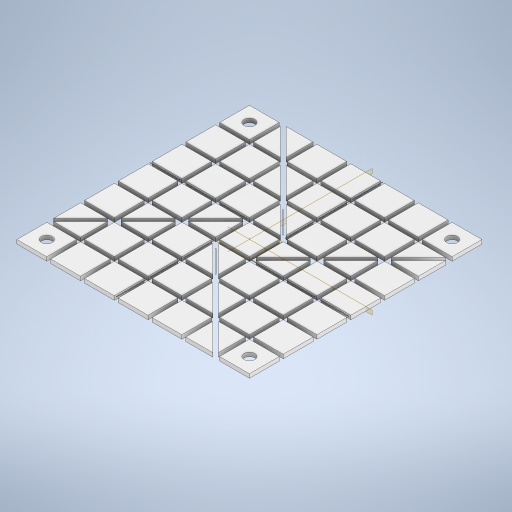
# Autodesk Inventor part: Flasher2
Saved by Autodesk Inventor 2024 (Build 280153000, 153)
## iProperties
Created: 2023-02-28
Part Number: Flasher2
Material: ABS Plastic
Document SubType Name: Modeling
Designer: byrne
Density: 1.06 g/cm^3
Appearance: Smooth - White
Author: byrne
Autodesk Inventor part; units mm, degrees
ref_plane "YZ Plane" through (0, 0, 0) normal (1, 0, 0) x (0, 1, 0)
ref_plane "XZ Plane" through (0, 0, 0) normal (0, 1, 0) x (-1, 0, 0)
ref_plane "XY Plane" through (0, 0, 0) normal (0, 0, 1) x (1, 0, 0)
sketch "Sketch1" plane through (0, 0, 0) normal (0, 1, 0) x (-1, 0, 0)
  line L0 (0, 0) -> (95.25, 0) construction
  line L1 (95.25, 0) -> (95.25, -95.25) construction
  line L2 (95.25, -95.25) -> (0, -95.25)
  line L3 (0, -95.25) -> (0, 0)
  line L4 (54.4286, -40.8214) -> (40.8214, -40.8214)
  line L5 (40.8214, -40.8214) -> (40.8214, -54.4286)
  line L6 (40.8214, -54.4286) -> (54.4286, -54.4286)
  line L7 (54.4286, -54.4286) -> (54.4286, -40.8214)
  line L8 (54.4286, -54.4286) -> (95.25, -13.6071)
  line L9 (40.8214, -54.4286) -> (81.6429, -95.25)
  line L10 (40.8214, -40.8214) -> (0, -81.6429)
  line L11 (54.4286, -40.8214) -> (13.6071, 0)
  line L12 (40.8214, -40.8214) -> (0, -40.8214)
  line L13 (40.8214, -54.4286) -> (40.8214, -95.25)
  line L14 (54.4286, -54.4286) -> (95.25, -54.4286)
  line L15 (54.4286, -40.8214) -> (54.4286, 0)
  line L16 (81.6429, -13.6071) -> (95.25, -13.6071)
  line L17 (81.6429, -13.6071) -> (81.6429, 0)
  line L18 (81.6429, -81.6429) -> (95.25, -81.6429)
  line L19 (81.6429, -81.6429) -> (81.6429, -95.25)
  line L20 (95.25, -81.6429) -> (95.25, -95.25)
  line L21 (95.25, -95.25) -> (81.6429, -95.25)
  line L22 (95.25, -13.6071) -> (95.25, 0)
  line L23 (95.25, 0) -> (81.6429, 0)
  line L24 (13.6071, 0) -> (0, 0)
  line L25 (0, -13.6071) -> (13.6071, -13.6071)
  line L26 (40.8214, -68.0357) -> (0, -68.0357)
  line L27 (40.8214, -54.4286) -> (0, -54.4286)
  line L28 (13.6071, -40.8214) -> (13.6071, -95.25)
  line L29 (40.8214, -81.6429) -> (0, -81.6429)
  line L30 (27.2143, -40.8214) -> (27.2143, -95.25)
  line L31 (41.3827, -41.3827) -> (1.9163, -80.8491)
  line L32 (1.9163, -80.8491) -> (40.8214, -80.8491)
  line L33 (40.2602, -40.2602) -> (-1.9163, -82.4366)
  line L34 (-1.9163, -82.4366) -> (40.8214, -82.4366)
  line L35 (40.8214, -68.8295) -> (0, -68.8295)
  line L36 (40.8214, -67.242) -> (0, -67.242)
  line L37 (26.4205, -40.8214) -> (26.4205, -95.25)
  line L38 (28.008, -40.8214) -> (28.008, -95.25)
  line L39 (40.0277, -54.4286) -> (40.0277, -95.25)
  line L40 (40.8214, -55.2223) -> (0, -55.2223)
  line L41 (40.8214, -53.6348) -> (0, -53.6348)
  line L42 (40.0277, -40.8214) -> (40.0277, -54.4286)
  line L43 (40.8214, -41.6152) -> (0, -41.6152)
  line L44 (14.4009, -40.8214) -> (14.4009, -95.25)
  line L45 (12.8134, -40.8214) -> (12.8134, -95.25)
  line L46 (0.7938, -95.25) -> (0.7937, -0.7938)
  line L47 (0.7937, -0.7938) -> (13.2784, -0.7938)
  line L48 (13.2784, -0.7938) -> (53.8673, -41.3827)
  line L49 (95.25, -94.4562) -> (0, -94.4562)
  line L50 (54.4286, -41.6152) -> (40.8214, -41.6152)
  line L51 (41.6152, -40.8214) -> (41.6152, -54.4286)
  line L52 (40.8214, -53.6348) -> (54.4286, -53.6348)
  line L53 (53.6348, -54.4286) -> (53.6348, -40.8214)
  circle A0 centre (6.8036, -88.4464) radius 2.159
  point P0 (27.2143, 0)
  point P1 (40.8214, 0)
  point P2 (68.0357, 0)
  point P3 (27.2143, -13.6071)
  point P4 (40.8214, -13.6071)
  point P5 (54.4286, -13.6071)
  point P6 (68.0357, -13.6071)
  point P7 (0, -27.2143)
  point P8 (13.6071, -27.2143)
  point P9 (27.2143, -27.2143)
  point P10 (40.8214, -27.2143)
  point P11 (54.4286, -27.2143)
  point P12 (68.0357, -27.2143)
  point P13 (81.6429, -27.2143)
  point P14 (95.25, -27.2143)
  point P15 (68.0357, -40.8214)
  point P16 (81.6429, -40.8214)
  point P17 (95.25, -40.8214)
  point P18 (13.6071, -54.4286)
  point P19 (27.2143, -54.4286)
  point P20 (68.0357, -54.4286)
  point P21 (81.6429, -54.4286)
  point P22 (13.6071, -68.0357)
  point P23 (27.2143, -68.0357)
  point P24 (54.4286, -68.0357)
  point P25 (68.0357, -68.0357)
  point P26 (81.6429, -68.0357)
  point P27 (95.25, -68.0357)
  point P28 (13.6071, -81.6429)
  point P29 (27.2143, -81.6429)
  point P30 (54.4286, -81.6429)
  point P31 (68.0357, -81.6429)
  point P32 (95.25, -81.6429)
  point P33 (0, -95.25)
  point P34 (54.4286, -95.25)
  point P35 (68.0357, -95.25)
  point P36 (53.6348, -53.6348)
  point P37 (53.6348, -41.6152)
  point P38 (41.6152, -41.6152)
  point P39 (41.6152, -53.6348)
  point P40 (0.7937, -55.2223)
  point P41 (0.7937, -67.242)
  point P42 (12.8134, -67.242)
  point P43 (12.8134, -55.2223)
  point P44 (0.7937, -41.6152)
  point P45 (0.7937, -53.6348)
  point P46 (12.8134, -53.6348)
  point P47 (12.8134, -41.6152)
  point P48 (0.7937, -68.8295)
  point P49 (0.7937, -79.7266)
  point P50 (11.6909, -68.8295)
  point P51 (12.8134, -80.8491)
  point P52 (12.8134, -69.952)
  point P53 (0.7937, -94.4562)
  point P54 (12.8134, -94.4562)
  point P55 (12.8134, -82.4366)
  point P56 (0.7937, -82.4366)
  point P57 (14.4009, -94.4562)
  point P58 (26.4205, -94.4562)
  point P59 (26.4205, -82.4366)
  point P60 (14.4009, -82.4366)
  point P61 (14.4009, -68.8295)
  point P62 (14.4009, -80.8491)
  point P63 (26.4205, -80.8491)
  point P64 (26.4205, -68.8295)
  point P65 (26.4205, -67.242)
  point P66 (26.4205, -56.3449)
  point P67 (15.5234, -67.242)
  point P68 (14.4009, -55.2223)
  point P69 (14.4009, -66.1194)
  point P70 (25.298, -55.2223)
  point P71 (14.4009, -41.6152)
  point P72 (14.4009, -53.6348)
  point P73 (26.4205, -53.6348)
  point P74 (26.4205, -41.6152)
  point P75 (38.9051, -41.6152)
  point P76 (28.008, -41.6152)
  point P77 (28.008, -52.5123)
  point P78 (40.0277, -53.6348)
  point P79 (40.0277, -42.7377)
  point P80 (29.1306, -53.6348)
  point P81 (40.0277, -55.2223)
  point P82 (28.008, -55.2223)
  point P83 (28.008, -67.242)
  point P84 (40.0277, -67.242)
  point P85 (40.0277, -80.8491)
  point P86 (40.0277, -68.8295)
  point P87 (28.008, -68.8295)
  point P88 (28.008, -80.8491)
  point P89 (28.008, -94.4562)
  point P90 (40.0277, -94.4562)
  point P91 (40.0277, -82.4366)
  point P92 (28.008, -82.4366)
  dimension "d0" = 95.25
  dimension "d1" = 95.25
  dimension "d4" = 13.6071
  dimension "d7" = 13.6071
  dimension "d10" = 0.7937
  dimension "d11" = 0.7937
  dimension "d12" = 0.7937
  dimension "d13" = 0.7937
  dimension "d14" = 0.7937
  dimension "d15" = 0.7937
  dimension "d16" = 0.7937
  dimension "d17" = 0.7937
  dimension "d18" = 0.7937
  dimension "d19" = 0.7937
  dimension "d20" = 0.7937
  dimension "d21" = 0.7937
  dimension "d22" = 0.7937
  dimension "d23" = 0.7937
  dimension "d24" = 0.7937
  dimension "d25" = 0.7937
  dimension "d26" = 0.7937
  dimension "d27" = 0.7937
  dimension "d28" = 0.7937
  dimension "d36" = 4.318
  dimension "d37" = 6.8036
  dimension "d38" = 6.8036
  constraints: 108 end point, 20 parallel, 7 horizontal, 6 perpendicular, 6 vertical, 3 collinear, 2 point on line, 1 centre point, 67 other
  measures "d0" distance of L1.end L2.end
  measures "d1" distance of L0.end L1.end
  measures "d4" distance of L0.start L11.end
  measures "d7" distance of L0.start L25.start
  measures "d10" distance between parallel lines of L10 L31
  measures "d11" distance between parallel lines of L10 L33
  measures "d12" distance between parallel lines of L26 L35
  measures "d13" distance between parallel lines of L26 L36
  measures "d14" distance between parallel lines of L30 L37
  measures "d15" distance between parallel lines of L30 L38
  measures "d16" distance between parallel lines of L13 L39
  measures "d17" distance between parallel lines of L27 L40
  measures "d18" distance between parallel lines of L27 L41
  measures "d19" distance between parallel lines of L5 L42
  measures "d20" distance between parallel lines of L12 L43
  measures "d21" distance between parallel lines of L28 L44
  measures "d22" distance between parallel lines of L28 L45
  measures "d23" distance between parallel lines of L3 L46
  measures "d24" distance between parallel lines of L2 L49
  measures "d25" distance between parallel lines of L4 L50
  measures "d26" distance between parallel lines of L5 L51
  measures "d27" distance between parallel lines of L6 L52
  measures "d28" distance between parallel lines of L7 L53
  measures "d36" diameter of A0
  measures "d37" distance from line of L2 A0.centre
  measures "d38" distance from line of A0.centre L3
extrude "Extrusion1" add sketch "Sketch1" along normal blind 1.5875 contours L51 L50 L53 L52
extrude "Extrusion2" add sketch "Sketch1" along normal blind 1.5875 contours L49 L38 L34 L39 | L41 L31 L42 | L39 L36 L38 L40 | L49 L44 L34 L37 | L32 L38 L35 L39 | L33 L38 L43 | L36 L31 L37 | L33 L44 L40 | L49 L46 L34 L45 | L32 L44 L35 L37 | L41 L44 L43 L37 | L33 L46 L35 | L45 L32 L31 | L36 L46 L40 L45 | L41 L46 L43 L45
ref_plane "Work Plane1" through (-47.625, 0, -41.6152) normal (1, 0, 0) x (0, 0, -1)
ref_plane "Work Plane2" through (-53.6348, 0, -47.625) normal (0, 0, 1) x (1, 0, 0)
pattern_circular "Circular Pattern1" count 4 over 360 about axis through (-47.625, 0, -47.625) along (0, -1, 0) of "Extrusion2"
sketch "Sketch3" plane through (0, 1.5875, 0) normal (0, 1, 0) x (1, 0, 0)
  line L0 (-40.9484, 94.3927) -> (-40.6944, 94.3927)
  line L1 (-40.6944, 55.2767) -> (-40.9484, 55.2767)
  line L2 (-41.6152, 94.4563) -> (-53.6348, 94.4563) projected
  line L3 (-40.0277, 94.4562) -> (-40.0277, 82.4366) projected
  line L4 (-41.6152, 94.4563) -> (-40.0277, 94.4562)
  line L5 (-40.9484, 82.4366) -> (-40.6944, 82.4366)
  line L6 (-53.6348, 82.4366) -> (-41.6152, 82.4366) projected
  line L7 (-40.9484, 80.8491) -> (-40.6944, 80.8491)
  line L8 (-41.6152, 80.8491) -> (-53.6348, 80.8491) projected
  line L9 (-40.9484, 68.8295) -> (-40.6944, 68.8295)
  line L10 (-40.9484, 67.242) -> (-40.6944, 67.242)
  line L11 (-53.6348, 68.8295) -> (-41.6152, 68.8295) projected
  line L12 (-41.6152, 67.242) -> (-52.5123, 67.242) projected
  line L13 (-40.6944, 94.3927) -> (-40.6944, 82.4366)
  line L14 (-40.9484, 82.4366) -> (-40.9484, 94.3927)
  line L15 (-40.6944, 80.8491) -> (-40.6944, 68.8295)
  line L16 (-40.6944, 67.242) -> (-40.6944, 55.2767)
  line L17 (-40.9484, 55.2767) -> (-40.9484, 67.242)
  line L18 (-40.9484, 68.8295) -> (-40.9484, 80.8491)
  line L19 (-41.6152, 53.6348) -> (-53.6348, 53.6348) projected
  line L20 (-41.6152, 41.6152) -> (-41.6152, 53.6348) projected
  line L21 (-55.2767, 54.5556) -> (-55.2767, 54.3016)
  line L22 (-68.8295, 54.3016) -> (-68.8295, 54.5556)
  line L23 (-67.242, 54.3016) -> (-67.242, 54.5556)
  line L24 (-67.242, 54.5556) -> (-55.2767, 54.5556)
  line L25 (-55.2767, 54.3016) -> (-67.242, 54.3016)
  line L26 (-94.3927, 54.3016) -> (-94.3927, 54.5556)
  line L27 (-94.4563, 53.6348) -> (-94.4562, 55.2223)
  line L28 (-80.8491, 54.5556) -> (-68.8295, 54.5556)
  line L29 (-68.8295, 54.3016) -> (-80.8491, 54.3016)
  line L30 (-80.8491, 54.3016) -> (-80.8491, 54.5556)
  line L31 (-82.4366, 54.3016) -> (-94.3927, 54.3016)
  line L32 (-94.3927, 54.5556) -> (-82.4366, 54.5556)
  line L33 (-82.4366, 54.3016) -> (-82.4366, 54.5556)
  line L34 (-54.5556, 39.9733) -> (-54.3016, 39.9733)
  line L35 (-54.3016, 26.4205) -> (-54.5556, 26.4205)
  line L36 (-54.3016, 28.008) -> (-54.5556, 28.008)
  line L37 (-54.5556, 28.008) -> (-54.5556, 39.9733)
  line L38 (-54.3016, 39.9733) -> (-54.3016, 28.008)
  line L39 (-54.3016, 0.8573) -> (-54.5556, 0.8573)
  line L40 (-53.6348, 0.7937) -> (-55.2223, 0.7937)
  line L41 (-54.5556, 14.4009) -> (-54.5556, 26.4205)
  line L42 (-54.3016, 26.4205) -> (-54.3016, 14.4009)
  line L43 (-54.3016, 14.4009) -> (-54.5556, 14.4009)
  line L44 (-54.3016, 12.8134) -> (-54.3016, 0.8573)
  line L45 (-54.5556, 0.8573) -> (-54.5556, 12.8134)
  line L46 (-54.3016, 12.8134) -> (-54.5556, 12.8134)
  line L47 (-39.9733, 40.6944) -> (-39.9733, 40.9484)
  line L48 (-26.4205, 40.9484) -> (-26.4205, 40.6944)
  line L49 (-28.008, 40.9484) -> (-28.008, 40.6944)
  line L50 (-28.008, 40.6944) -> (-39.9733, 40.6944)
  line L51 (-39.9733, 40.9484) -> (-28.008, 40.9484)
  line L52 (-0.8573, 40.9484) -> (-0.8573, 40.6944)
  line L53 (-0.7937, 41.6152) -> (-0.7937, 40.0277)
  line L54 (-14.4009, 40.6944) -> (-26.4205, 40.6944)
  line L55 (-26.4205, 40.9484) -> (-14.4009, 40.9484)
  line L56 (-14.4009, 40.9484) -> (-14.4009, 40.6944)
  line L57 (-12.8134, 40.9484) -> (-0.8573, 40.9484)
  line L58 (-0.8573, 40.6944) -> (-12.8134, 40.6944)
  line L59 (-12.8134, 40.9484) -> (-12.8134, 40.6944)
  point P0 (0, 0)
  point P1 (-40.8214, 94.4563)
  point P2 (-40.8214, 94.3927)
  point P3 (-40.8214, 67.242)
  point P4 (-40.8214, 80.8491)
  point P5 (-47.625, 47.625)
  point P6 (-47.625, 53.6348)
  point P7 (-41.6152, 47.625)
  point P8 (-67.242, 54.4286)
  point P9 (-94.3927, 54.4286)
  point P10 (-94.4563, 54.4286)
  point P11 (-80.8491, 54.4286)
  point P12 (-54.4286, 28.008)
  point P13 (-54.4286, 0.8573)
  point P14 (-54.4286, 0.7937)
  point P15 (-54.4286, 14.4009)
  point P16 (-28.008, 40.8214)
  point P17 (-0.8573, 40.8214)
  point P18 (-0.7937, 40.8214)
  point P19 (-14.4009, 40.8214)
  dimension "d39" = 39.116
  dimension "d40" = 0.254
  dimension "d41" = 0.0635
  dimension "d44" = 360
  constraints: 104 end point, 15 perpendicular, 12 parallel, 6 midpoint, 4 collinear, 4 vertical alignment, 2 horizontal, 1 horizontal alignment, 125 other
  measures "d39" distance of L0.end L1.start
  measures "d40" distance of L0.start L0.end
  measures "d41" distance between parallel lines of L2 L0
sketch "Sketch4" plane through (0, 1.5875, 0) normal (0, 1, 0) x (1, 0, 0)
  line L0 (-56.8318, 52.2049) -> (-56.6522, 52.0253)
  line L1 (-56.6522, 52.0253) -> (-65.6325, 43.0451)
  line L2 (-65.6325, 43.0451) -> (-65.8121, 43.2247)
  line L3 (-65.8121, 43.2247) -> (-56.8318, 52.2049)
  line L4 (-67.242, 42.7377) -> (-56.3449, 53.6348) projected
  line L5 (-67.242, 53.6348) -> (-67.242, 42.7377) projected
  line L6 (-67.242, 53.6348) -> (-61.3219, 47.7148) construction
  line L7 (-55.2223, 52.5123) -> (-66.1194, 41.6152) projected
  line L8 (-61.7934, 48.1863) -> (-60.6709, 47.0637) construction
  line L9 (-61.3219, 47.7148) -> (-61.1423, 47.5352) construction
  line L10 (-52.0253, 38.5978) -> (-43.0451, 29.6175)
  line L11 (-43.2247, 29.4379) -> (-52.2049, 38.4182)
  line L12 (-43.0451, 29.6175) -> (-43.2247, 29.4379)
  line L13 (-52.2049, 38.4182) -> (-52.0253, 38.5978)
  line L14 (-38.5978, 43.2247) -> (-29.6175, 52.2049)
  line L15 (-29.4379, 52.0253) -> (-38.4182, 43.0451)
  line L16 (-29.6175, 52.2049) -> (-29.4379, 52.0253)
  line L17 (-38.4182, 43.0451) -> (-38.5978, 43.2247)
  line L18 (-43.2247, 56.6522) -> (-52.2049, 65.6325)
  line L19 (-52.0253, 65.8121) -> (-43.0451, 56.8318)
  line L20 (-52.2049, 65.6325) -> (-52.0253, 65.8121)
  line L21 (-43.0451, 56.8318) -> (-43.2247, 56.6522)
  point P0 (0, 0)
  point P1 (-61.2321, 47.625)
  point P2 (-47.625, 47.625)
  point P3 (-47.625, 47.625)
  point P4 (-47.5352, 34.1077)
  point P5 (-47.7148, 33.9281)
  point P6 (-34.1077, 47.7148)
  point P7 (-33.9281, 47.5352)
  point P8 (-47.7148, 61.1423)
  point P9 (-47.5352, 61.3219)
  dimension "d46" = 0.254
  dimension "d47" = 12.7
  dimension "d50" = 360
  constraints: 38 end point, 9 midpoint, 3 parallel, 3 perpendicular, 1 coincident, 1 point on line, 41 other
  measures "d46" distance of L0.start L0.end
  measures "d47" distance of L0.end L1.end
extrude "Extrusion3" add sketch "Sketch3" along normal blind 0.0508
ref_plane "Work Plane3" through (0, 0.7874, 0) normal (0, 1, 0) x (1, 0, 0)
extrude "Extrusion4" add sketch "Sketch4" against normal blind 0.0508 from surface at -0.8001
equation "\"d0\" = d1"
equation "\"d4\" = d7"
equation "\"d7\" = 0.142857 * d1"
equation "\"d37\" = 0.5 * d4"
equation "\"d38\" = d37"
body "Solid1"
